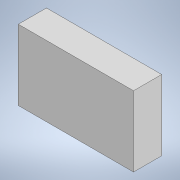
# Autodesk Inventor part: Coté
Saved by Autodesk Inventor 2020 (Build 240168000, 168)
## iProperties
Created: 2019-11-07
Part Number: Coté
Material: Générique
Document SubType Name: Modeling
Designer: erwan
Density: 1 g/cm^3
Appearance: Par défaut
Author: erwan
Autodesk Inventor part; units mm, degrees
ref_plane "YZ Plane" through (0, 0, 0) normal (1, 0, 0) x (0, 1, 0)
ref_plane "XZ Plane" through (0, 0, 0) normal (0, 1, 0) x (-1, 0, 0)
ref_plane "XY Plane" through (0, 0, 0) normal (0, 0, 1) x (1, 0, 0)
sketch "Esquisse1" plane through (0, 0, 0) normal (0, 1, 0) x (-1, 0, 0)
  line L0 (0, 0) -> (90, 0)
  line L1 (90, 0) -> (90, -22)
  line L2 (90, -22) -> (0, -22)
  line L3 (0, -22) -> (0, 0)
  line L4 (75.7217, 0) -> (53.9694, 0)
  line L5 (53.9694, 0) -> (53.9694, 22)
  line L6 (53.9694, 22) -> (75.7217, 22)
  line L7 (75.7217, 22) -> (75.7217, 0)
  dimension "d0" = 90
  dimension "d1" = 22
  dimension "d4" = 22
  constraints: 16 end point, 4 parallel, 2 horizontal, 2 perpendicular, 1 point on line
  measures "d0" distance of L1.end L2.end
  measures "d1" distance of L0.end L1.end
  measures "d4" distance between parallel lines of L6 L0
extrude "Extrusion1" add sketch "Esquisse1" along normal blind 55 contours L0 L1 L2 L3
